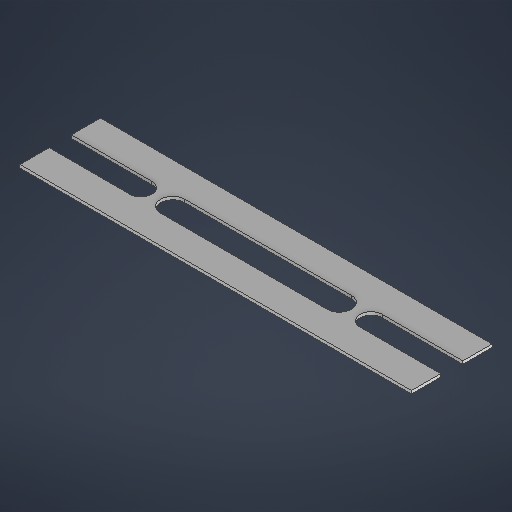
# Autodesk Inventor part: Galvo Spacer Y
Saved by Autodesk Inventor 2025 (Build 290162000, 162)
## iProperties
Created: 2024-07-08
Part Number: Galvo Spacer Y
Material: Generic
Document SubType Name: Modeling
Designer: mayhe
Density: 1 g/cm^3
Appearance: Default
Author: mayhe
Autodesk Inventor part; units mm, degrees
ref_plane "YZ Plane" through (0, 0, 0) normal (1, 0, 0) x (0, 1, 0)
ref_plane "XZ Plane" through (0, 0, 0) normal (0, 1, 0) x (-1, 0, 0)
ref_plane "XY Plane" through (0, 0, 0) normal (0, 0, 1) x (1, 0, 0)
sketch "Sketch5" plane through (0, 0, 0) normal (0, 0, 1) x (1, 0, 0)
  line L0 (68.6, -0.5) -> (-28.6, -0.5)
  line L1 (-28.6, -0.5) -> (-28.6, 0.25)
  line L2 (-28.6, 0.25) -> (68.6, 0.25)
  line L3 (68.6, 0.25) -> (68.6, -0.5)
  line L4 (68.6, -0.5) -> (-28.6, 0.25) construction
  line L5 (-28.6, -0.5) -> (68.6, 0.25) construction
  point P0 (20, -0.125)
  dimension "d83" = 97.2
  dimension "d84" = 0.75
  constraints: 12 end point, 2 midpoint, 2 parallel, 1 horizontal, 1 perpendicular
  measures "d83" distance of L1.end L2.end
  measures "d84" distance of L0.end L1.end
extrude "Extrusion5" add sketch "Sketch5" along normal mid plane 20
sketch "Sketch7" plane through (-28.6, -0.5, 10) normal (0, -1, 0) x (1, 0, 0)
  circle A0 centre (77.2, -10) radius 2.75
  circle A1 centre (20, -10) radius 2.75
  line L0 (0, 0) -> (97.2, 0) projected
  line L1 (97.2, -20) -> (97.2, 0) projected
  line L2 (0, -20) -> (0, 0) projected
  line L3 (77.2, -12.75) -> (97.2, -12.75)
  line L4 (97.2, -12.75) -> (97.2, -7.25)
  line L5 (97.2, -7.25) -> (77.2, -7.25)
  line L6 (77.2, -7.25) -> (77.2, -12.75)
  line L7 (20, -12.75) -> (0, -12.75)
  line L8 (0, -12.75) -> (0, -7.25)
  line L9 (0, -7.25) -> (20, -7.25)
  line L10 (20, -7.25) -> (20, -12.75)
  arc A2 (27.94, -7) -> (27.94, -13) centre (27.94, -10) ccw
  line L11 (48.6, 0) -> (48.6, -20)
  line L12 (97.2, -20) -> (0, -20) projected
  line L13 (27.94, -7) -> (48.6, -7)
  line L14 (27.94, -13) -> (48.6, -13)
  line L15 (27.94, -13) -> (48.6, -13) construction
  arc A3 (69.26, -13) -> (69.26, -7) centre (69.26, -10) ccw
  line L16 (69.26, -7) -> (48.6, -7)
  line L17 (69.26, -13) -> (48.6, -13)
  line L18 (69.26, -13) -> (48.6, -13) construction
  point P0 (28.6, -10)
  point P1 (0, -10)
  point P2 (20, -7.25)
  point P3 (77.2, -7.25)
  dimension "d85" = 5.5
  dimension "d86" = 5.5
  dimension "d87" = 10
  dimension "d88" = 20
  dimension "d89" = 20
  dimension "d90" = 10
  dimension "d93" = 6
  dimension "d94" = 27.94
  constraints: 30 end point, 6 point on line, 4 parallel, 4 point on circle, 3 horizontal, 3 midpoint, 3 perpendicular, 3 symmetric about line, 2 centre point, 1 collinear, 1 tangent, 7 other
  measures "d87" distance from line of L0 point (77.2, -10)
  measures "d88" distance from line of L1 point (77.2, -10)
  measures "d89" distance of point (0, -10) point (20, -10)
  measures "d90" distance from line of L0 point (20, -10)
  measures "d93" diameter of A2
  measures "d94" distance from line of L2 A2.centre
extrude "Extrusion7" cut sketch "Sketch7" against normal blind 20 contours A0 L6 | A0 L5 L1 L3 | L6 A0 | L16 A3 L17 L11 | L11 L14 A2 L13 | L9 A1 L7 L2 | L10 A1 | A1 L10
body "Solid3"
